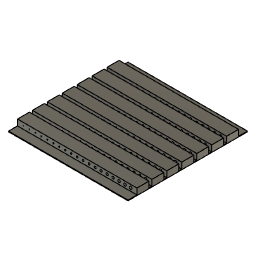
Test strip v1 (Autodesk Fusion 360 design; units mm, degrees)
Autodesk Fusion 360 part; units mm, degrees
sketch "Sketch1" plane through (0, 0, 0) normal (0, 0, 1) x (1, 0, 0)
  line L0 (50, 50) -> (-50, 50)
  line L1 (-50, 50) -> (-50, -50)
  line L2 (-50, -50) -> (50, -50)
  line L3 (50, -50) -> (50, 50)
  line L4 (50, 50) -> (-50, -50) construction
  line L5 (-50, 50) -> (50, -50) construction
  line L6 (0, 0) -> (-50, 0) construction
  line L7 (-25, 0) -> (-25, 50) construction
  line L8 (-50, 50) -> (-25, 0) construction
  line L9 (-25, 50) -> (-50, 0) construction
  line L10 (-37.5, 25) -> (-37.5, 50) construction
  line L11 (-37.5, 25) -> (-37.5, -50) construction
  line L12 (-25, 0) -> (-25, -50) construction
  line L13 (-25, 0) -> (0, 0) construction
  line L14 (-12.5, 0) -> (-12.5, 50) construction
  line L15 (-12.5, 0) -> (-12.5, -50) construction
  line L16 (0, 0) -> (0, -50) construction
  line L17 (0, 0) -> (0, 50) construction
  line L18 (0, 0) -> (50, 0) construction
  line L19 (25, 0) -> (25, 50) construction
  line L20 (25, 0) -> (25, -50) construction
  line L21 (0, 0) -> (25, 0) construction
  line L22 (12.5, 0) -> (12.5, -50) construction
  line L23 (12.5, 0) -> (12.5, 50) construction
  line L24 (25, 0) -> (50, 0) construction
  line L25 (37.5, 0) -> (37.5, -50) construction
  line L26 (37.5, 0) -> (37.5, 50) construction
  line L27 (-50, 0) -> (-50, 50) construction
  line L28 (-50, 25) -> (50, 25) construction
  line L29 (-50, 50) -> (-50, 25) construction
  line L30 (-50, 37.5) -> (50, 37.5) construction
  line L31 (-50, 25) -> (-50, 0) construction
  line L32 (-50, 12.5) -> (50, 12.5) construction
  line L33 (-50, -50) -> (-50, 0) construction
  line L34 (-50, -25) -> (50, -25) construction
  line L35 (-50, 0) -> (-50, -25) construction
  line L36 (-50, -12.5) -> (50, -12.5) construction
  line L37 (-50, -25) -> (-50, -50) construction
  line L38 (-50, -37.5) -> (50, -37.5) construction
  line L39 (-25, 42.5) -> (-50, 42.5)
  line L40 (-50, 42.5) -> (-50, 32.5)
  line L41 (-50, 32.5) -> (-25, 32.5)
  line L42 (-25, 32.5) -> (-25, 42.5)
  line L43 (-25, 42.5) -> (-50, 32.5) construction
  line L44 (-50, 42.5) -> (-25, 32.5) construction
  line L45 (-25, 30) -> (-50, 30)
  line L46 (-50, 30) -> (-50, 20)
  line L47 (-50, 20) -> (-25, 20)
  line L48 (-25, 20) -> (-25, 30)
  line L49 (-25, 30) -> (-50, 20) construction
  line L50 (-50, 30) -> (-25, 20) construction
  line L51 (-25, 17.5) -> (-50, 17.5)
  line L52 (-50, 17.5) -> (-50, 7.5)
  line L53 (-50, 7.5) -> (-25, 7.5)
  line L54 (-25, 7.5) -> (-25, 17.5)
  line L55 (-25, 17.5) -> (-50, 7.5) construction
  line L56 (-50, 17.5) -> (-25, 7.5) construction
  line L57 (-25, 5) -> (-50, 5)
  line L58 (-50, 5) -> (-50, -5)
  line L59 (-50, -5) -> (-25, -5)
  line L60 (-25, -5) -> (-25, 5)
  line L61 (-25, 5) -> (-50, -5) construction
  line L62 (-50, 5) -> (-25, -5) construction
  line L63 (-25, -7.5) -> (-50, -7.5)
  line L64 (-50, -7.5) -> (-50, -17.5)
  line L65 (-50, -17.5) -> (-25, -17.5)
  line L66 (-25, -17.5) -> (-25, -7.5)
  line L67 (-25, -7.5) -> (-50, -17.5) construction
  line L68 (-50, -7.5) -> (-25, -17.5) construction
  line L69 (-25, -20) -> (-50, -20)
  line L70 (-50, -20) -> (-50, -30)
  line L71 (-50, -30) -> (-25, -30)
  line L72 (-25, -30) -> (-25, -20)
  line L73 (-25, -20) -> (-50, -30) construction
  line L74 (-50, -20) -> (-25, -30) construction
  line L75 (-25, -32.5) -> (-50, -32.5)
  line L76 (-50, -32.5) -> (-50, -42.5)
  line L77 (-50, -42.5) -> (-25, -42.5)
  line L78 (-25, -42.5) -> (-25, -32.5)
  line L79 (-25, -32.5) -> (-50, -42.5) construction
  line L80 (-50, -32.5) -> (-25, -42.5) construction
  line L81 (-25, 32.5) -> (0, 32.5)
  line L82 (0, 32.5) -> (0, 42.5)
  line L83 (0, 42.5) -> (-25, 42.5)
  line L84 (-25, 42.5) -> (-25, 32.5)
  line L85 (-25, 20) -> (0, 20)
  line L86 (0, 20) -> (0, 30)
  line L87 (-25, 30) -> (-25, 20)
  line L88 (0, 30) -> (-25, 30)
  line L89 (-25, 7.5) -> (0, 7.5)
  line L90 (0, 7.5) -> (0, 17.5)
  line L91 (-25, 17.5) -> (-25, 7.5)
  line L92 (0, 17.5) -> (-25, 17.5)
  line L93 (-25, -5) -> (0, -5)
  line L94 (0, -5) -> (0, 5)
  line L95 (-25, 5) -> (-25, -5)
  line L96 (0, 5) -> (-25, 5)
  line L97 (-25, -17.5) -> (0, -17.5)
  line L98 (0, -17.5) -> (0, -7.5)
  line L99 (-25, -7.5) -> (-25, -17.5)
  line L100 (0, -7.5) -> (-25, -7.5)
  line L101 (-25, -30) -> (0, -30)
  line L102 (0, -30) -> (0, -20)
  line L103 (-25, -20) -> (-25, -30)
  line L104 (0, -20) -> (-25, -20)
  line L105 (-25, -42.5) -> (0, -42.5)
  line L106 (0, -42.5) -> (0, -32.5)
  line L107 (-25, -32.5) -> (-25, -42.5)
  line L108 (0, -32.5) -> (-25, -32.5)
  line L109 (0, 32.5) -> (25, 32.5)
  line L110 (25, 32.5) -> (25, 42.5)
  line L111 (25, 42.5) -> (0, 42.5)
  line L112 (0, 42.5) -> (0, 32.5)
  line L113 (0, 20) -> (25, 20)
  line L114 (25, 20) -> (25, 30)
  line L115 (0, 30) -> (0, 20)
  line L116 (25, 30) -> (0, 30)
  line L117 (0, 7.5) -> (25, 7.5)
  line L118 (25, 7.5) -> (25, 17.5)
  line L119 (0, 17.5) -> (0, 7.5)
  line L120 (25, 17.5) -> (0, 17.5)
  line L121 (0, -5) -> (25, -5)
  line L122 (25, -5) -> (25, 5)
  line L123 (0, 5) -> (0, -5)
  line L124 (25, 5) -> (0, 5)
  line L125 (0, -17.5) -> (25, -17.5)
  line L126 (25, -17.5) -> (25, -7.5)
  line L127 (0, -7.5) -> (0, -17.5)
  line L128 (25, -7.5) -> (0, -7.5)
  line L129 (0, -30) -> (25, -30)
  line L130 (25, -30) -> (25, -20)
  line L131 (0, -20) -> (0, -30)
  line L132 (25, -20) -> (0, -20)
  line L133 (0, -42.5) -> (25, -42.5)
  line L134 (25, -42.5) -> (25, -32.5)
  line L135 (0, -32.5) -> (0, -42.5)
  line L136 (25, -32.5) -> (0, -32.5)
  line L137 (25, 32.5) -> (50, 32.5)
  line L138 (50, 32.5) -> (50, 42.5)
  line L139 (50, 42.5) -> (25, 42.5)
  line L140 (25, 42.5) -> (25, 32.5)
  line L141 (25, 20) -> (50, 20)
  line L142 (50, 20) -> (50, 30)
  line L143 (25, 30) -> (25, 20)
  line L144 (50, 30) -> (25, 30)
  line L145 (25, 7.5) -> (50, 7.5)
  line L146 (50, 7.5) -> (50, 17.5)
  line L147 (25, 17.5) -> (25, 7.5)
  line L148 (50, 17.5) -> (25, 17.5)
  line L149 (25, -5) -> (50, -5)
  line L150 (50, -5) -> (50, 5)
  line L151 (25, 5) -> (25, -5)
  line L152 (50, 5) -> (25, 5)
  line L153 (25, -17.5) -> (50, -17.5)
  line L154 (50, -17.5) -> (50, -7.5)
  line L155 (25, -7.5) -> (25, -17.5)
  line L156 (50, -7.5) -> (25, -7.5)
  line L157 (25, -30) -> (50, -30)
  line L158 (50, -30) -> (50, -20)
  line L159 (25, -20) -> (25, -30)
  line L160 (50, -20) -> (25, -20)
  line L161 (25, -42.5) -> (50, -42.5)
  line L162 (50, -42.5) -> (50, -32.5)
  line L163 (25, -32.5) -> (25, -42.5)
  line L164 (50, -32.5) -> (25, -32.5)
  point P0 (-37.5, 37.5)
  point P1 (-37.5, 25)
  point P2 (-37.5, 12.5)
  point P3 (-37.5, 0)
  point P4 (-37.5, -12.5)
  point P5 (-37.5, -25)
  point P6 (-37.5, -37.5)
  dimension "d1" = 100
  dimension "d2" = 100
  dimension "d3" = 10
  dimension "d4" = 10
  dimension "d5" = 10
  dimension "d6" = 10
  dimension "d7" = 10
  dimension "d8" = 10
  dimension "d9" = 10
  dimension "d10" = 10
  dimension "d11" = 10
  dimension "d12" = 10
  dimension "d13" = 10
  dimension "d14" = 10
  dimension "d15" = 10
  dimension "d16" = 10
  dimension "d17" = 10
  dimension "d18" = 10
  dimension "d19" = 10
  dimension "d20" = 10
  dimension "d21" = 10
  dimension "d22" = 10
  dimension "d23" = 10
  dimension "d24" = 10
  dimension "d25" = 10
  dimension "d26" = 10
  dimension "d27" = 10
  dimension "d28" = 10
  dimension "d29" = 10
  dimension "d30" = 10
  constraint horizontal L0
  constraint perpendicular L0 L1
  constraint parallel L0 L2
  constraint parallel L1 L3
  constraint coincident L4 L6.start
  constraint coincident L5 L6.start
  constraint coincident L6.start L13.end
  constraint midpoint L1 L6.end
  constraint midpoint L6 L7.start
  constraint coincident L0 L7.end
  constraint perpendicular L0 L7
  constraint midpoint L8 P1
  constraint coincident L0 L10.end
  constraint perpendicular L0 L10
  constraint coincident L2 L11.end
  constraint perpendicular L2 L11
  constraint coincident L2 L12.end
  constraint perpendicular L2 L12
  constraint midpoint L13 L14.start
  constraint coincident L0 L14.end
  constraint perpendicular L0 L14
  constraint coincident L2 L15.end
  constraint perpendicular L2 L15
  constraint midpoint L2 L16.end
  constraint midpoint L0 L17.end
  constraint midpoint L3 L18.end
  constraint midpoint L18 L19.start
  constraint coincident L0 L19.end
  constraint perpendicular L0 L19
  constraint coincident L2 L20.end
  constraint perpendicular L2 L20
  constraint midpoint L21 L22.start
  constraint coincident L2 L22.end
  constraint perpendicular L2 L22
  constraint coincident L0 L23.end
  constraint perpendicular L0 L23
  constraint midpoint L24 L25.start
  constraint coincident L2 L25.end
  constraint perpendicular L2 L25
  constraint coincident L0 L26.end
  constraint perpendicular L0 L26
  constraint midpoint L27 L28.start
  constraint coincident L3 L28.end
  constraint perpendicular L3 L28
  constraint midpoint L29 L30.start
  constraint perpendicular L26 L30
  constraint midpoint L31 L32.start
  constraint coincident L3 L32.end
  constraint perpendicular L3 L32
  constraint midpoint L33 L34.start
  constraint coincident L3 L34.end
  constraint perpendicular L3 L34
  constraint midpoint L35 L36.start
  constraint coincident L3 L36.end
  constraint perpendicular L3 L36
  constraint midpoint L37 L38.start
  constraint coincident L3 L38.end
  constraint perpendicular L3 L38
  constraint horizontal L39
  constraint perpendicular L39 L40
  constraint parallel L39 L41
  constraint parallel L40 L42
  constraint coincident L43 P0
  constraint coincident L44 P0
  constraint midpoint L10 P0
  constraint horizontal L45
  constraint perpendicular L45 L46
  constraint parallel L45 L47
  constraint parallel L46 L48
  constraint coincident L49 P1
  constraint coincident L50 P1
  constraint coincident P1 L10.start
  constraint horizontal L51
  constraint perpendicular L51 L52
  constraint parallel L51 L53
  constraint parallel L52 L54
  constraint coincident L55 P2
  constraint coincident L56 P2
  constraint coincident L7 L51.start
  constraint coincident L32 P2
  constraint coincident L11 P2
  constraint horizontal L57
  constraint perpendicular L57 L58
  constraint parallel L57 L59
  constraint parallel L58 L60
  constraint coincident L61 P3
  constraint coincident L62 P3
  constraint coincident L11 P3
  constraint coincident L6 P3
  constraint horizontal L63
  constraint perpendicular L63 L64
  constraint parallel L63 L65
  constraint parallel L64 L66
  constraint coincident L67 P4
  constraint coincident L68 P4
  constraint midpoint L11 P4
  constraint horizontal L69
  constraint perpendicular L69 L70
  constraint parallel L69 L71
  constraint parallel L70 L72
  constraint coincident L73 P5
  constraint coincident L74 P5
  constraint coincident L34 P5
  constraint coincident L11 P5
  constraint horizontal L75
  constraint perpendicular L75 L76
  constraint parallel L75 L77
  constraint parallel L76 L78
  constraint coincident L79 P6
  constraint coincident L80 P6
  constraint coincident L38 P6
  constraint coincident L4 P6
  constraint horizontal L83
  constraint perpendicular L83 L84
  constraint parallel L81 L83
  constraint parallel L82 L84
  constraint horizontal L88
  constraint perpendicular L87 L88
  constraint parallel L85 L88
  constraint parallel L86 L87
  constraint horizontal L92
  constraint perpendicular L91 L92
  constraint parallel L89 L92
  constraint parallel L90 L91
  constraint horizontal L96
  constraint perpendicular L95 L96
  constraint parallel L93 L96
  constraint parallel L94 L95
  constraint horizontal L100
  constraint perpendicular L99 L100
  constraint parallel L97 L100
  constraint parallel L98 L99
  constraint horizontal L104
  constraint perpendicular L103 L104
  constraint parallel L101 L104
  constraint parallel L102 L103
  constraint horizontal L108
  constraint perpendicular L107 L108
  constraint parallel L105 L108
  constraint parallel L106 L107
  constraint horizontal L111
  constraint perpendicular L111 L112
  constraint parallel L109 L111
  constraint parallel L110 L112
  constraint horizontal L116
  constraint perpendicular L115 L116
  constraint parallel L113 L116
  constraint parallel L114 L115
  constraint horizontal L120
  constraint perpendicular L119 L120
  constraint parallel L117 L120
  constraint parallel L118 L119
  constraint horizontal L124
  constraint perpendicular L123 L124
  constraint parallel L121 L124
  constraint parallel L122 L123
  constraint horizontal L128
  constraint perpendicular L127 L128
  constraint parallel L125 L128
  constraint parallel L126 L127
  constraint horizontal L132
  constraint perpendicular L131 L132
  constraint parallel L129 L132
  constraint parallel L130 L131
  constraint horizontal L136
  constraint perpendicular L135 L136
  constraint parallel L133 L136
  constraint parallel L134 L135
  constraint horizontal L139
  constraint perpendicular L139 L140
  constraint parallel L137 L139
  constraint parallel L138 L140
  constraint horizontal L144
  constraint perpendicular L143 L144
  constraint parallel L141 L144
  constraint parallel L142 L143
  constraint horizontal L148
  constraint perpendicular L147 L148
  constraint parallel L145 L148
  constraint parallel L146 L147
  constraint horizontal L152
  constraint perpendicular L151 L152
  constraint parallel L149 L152
  constraint parallel L150 L151
  constraint horizontal L156
  constraint perpendicular L155 L156
  constraint parallel L153 L156
  constraint parallel L154 L155
  constraint horizontal L160
  constraint perpendicular L159 L160
  constraint parallel L157 L160
  constraint parallel L158 L159
  constraint horizontal L164
  constraint perpendicular L163 L164
  constraint parallel L161 L164
  constraint parallel L162 L163
  measures "d1" distance of L1.end L2.end
  measures "d2" distance of L0.end L1.end
  measures "d3" distance of L39.end L40.end
  measures "d4" distance of L45.end L46.end
  measures "d5" distance of L51.end L52.end
  measures "d6" distance of L57.end L58.end
  measures "d7" distance of L63.end L64.end
  measures "d8" distance of L69.end L70.end
  measures "d9" distance of L75.end L76.end
  measures "d10" distance of L41.end L39.start
  measures "d11" distance of L45.start L47.end
  measures "d12" distance of L51.start L53.end
  measures "d13" distance of L59.end L57.start
  measures "d14" distance of L65.end L63.start
  measures "d15" distance of L69.start L71.end
  measures "d16" distance of L75.start L77.end
  measures "d17" distance of L81.end L82.end
  measures "d18" distance of L86.end L85.end
  measures "d19" distance of L90.end L89.end
  measures "d20" distance of L93.end L94.end
  measures "d21" distance of L97.end L98.end
  measures "d22" distance of L102.end L101.end
  measures "d23" distance of L106.end L105.end
  measures "d24" distance of L109.end L110.end
  measures "d25" distance of L114.end L113.end
  measures "d26" distance of L118.end L117.end
  measures "d27" distance of L121.end L122.end
  measures "d28" distance of L125.end L126.end
  measures "d29" distance of L130.end L129.end
  measures "d30" distance of L134.end L133.end
extrude "Extrude1" add sketch "Sketch1" along normal blind 5 contours L3 L110 L137 L138 L139 L140 | L1 L39 L40 L41 L42 L84 | L82 L109 L110 L111 L112 L140 | L42 L81 L82 L83 L84 L112 | L3 L114 L141 L142 L143 L144 | L1 L45 L46 L47 L48 L87 | L86 L113 L114 L115 L116 L143 | L48 L85 L86 L87 L88 L115 | L3 L118 L145 L146 L147 L148 | L1 L51 L52 L53 L54 L91 | L90 L117 L118 L119 L120 L147 | L54 L89 L90 L91 L92 L119 | L3 L122 L149 L150 L151 L152 | L1 L57 L58 L59 L60 L95 | L94 L121 L122 L123 L124 L151 | L60 L93 L94 L95 L96 L123 | L3 L126 L153 L154 L155 L156 | L1 L63 L64 L65 L66 L99 | L98 L125 L126 L127 L128 L155 | L66 L97 L98 L99 L100 L127 | L3 L130 L157 L158 L159 L160 | L1 L69 L70 L71 L72 L103 | L102 L129 L130 L131 L132 L159 | L72 L101 L102 L103 L104 L131 | L3 L134 L161 L162 L163 L164 | L1 L75 L76 L77 L78 L107 | L106 L133 L134 L135 L136 L163 | L78 L105 L106 L107 L108 L135 makes body 1 at (-16.6667, -10.8333, 0) makes body 2 at (-16.6667, 39.1667, 0) makes body 3 at (16.6667, -1.6667, 0) makes body 4 at (-16.6667, -23.3333, 0) makes body 5 at (-16.6667, 26.6667, 0) makes body 6 at (-16.6667, 14.1667, 0) makes body 7 at (-16.6667, -35.8333, 0)
extrude "Extrude2" add sketch "Sketch1" against normal blind 0.5 bodies 1 2 3 4 5 6 7
hole "Hole1" at (-45, -42.5, 2.5) direction (0, 1, 0) diameter 0.5 end through all bodies 1
hole "Hole2" at (-40, -42.5, 2.5) direction (0, 1, 0) diameter 0.6 end through all bodies 1
hole "Hole3" at (-35, -42.5, 2.5) direction (0, 1, 0) diameter 0.7 end through all bodies 1
hole "Hole4" at (-30, -42.5, 2.5) direction (0, 1, 0) diameter 0.8 depth 85 tip angle 118 bodies 1
hole "Hole5" at (-25, -42.5, 2.5) direction (0, 1, 0) diameter 0.9 depth 85 tip angle 118 bodies 1
hole "Hole6" at (-20, -42.5, 2.5) direction (0, 1, 0) diameter 1 depth 85 tip angle 118 bodies 1
hole "Hole7" at (-15, -42.5, 2.5) direction (0, 1, 0) diameter 1.1 end through all bodies 1
hole "Hole8" at (-10, -42.5, 2.5) direction (0, 1, 0) diameter 1.2 depth 85 tip angle 118 bodies 1
hole "Hole9" at (-5, -42.5, 2.5) direction (0, 1, 0) diameter 1.3 depth 85 tip angle 118 bodies 1
hole "Hole10" at (0, -42.5, 2.5) direction (0, 1, 0) diameter 1.4 depth 85 tip angle 118 bodies 1
hole "Hole11" at (5, -42.5, 2.5) direction (0, 1, 0) diameter 1.5 depth 85 tip angle 118 bodies 1
hole "Hole12" at (10, -42.5, 2.5) direction (0, 1, 0) diameter 1.6 depth 85 tip angle 118 bodies 1
hole "Hole13" at (15, -42.5, 2.5) direction (0, 1, 0) diameter 1.7 end through all bodies 1
hole "Hole14" at (20, -42.5, 2.5) direction (0, 1, 0) diameter 1.8 depth 85 tip angle 118 bodies 1
hole "Hole15" at (25, -42.5, 2.5) direction (0, 1, 0) diameter 1.9 depth 85 tip angle 118 bodies 1
hole "Hole16" at (30, -42.5, 2.5) direction (0, 1, 0) diameter 2 depth 85 tip angle 118 bodies 1
hole "Hole17" at (35, -42.5, 2.5) direction (0, 1, 0) diameter 2.1 depth 85 tip angle 118 bodies 1
hole "Hole18" at (40, -42.5, 2.5) direction (0, 1, 0) diameter 2.2 depth 85 tip angle 118 bodies 1
hole "Hole19" at (44.7881, -42.5, 2.5) direction (0, 1, 0) diameter 2.3 depth 95 tip angle 118 bodies 1
